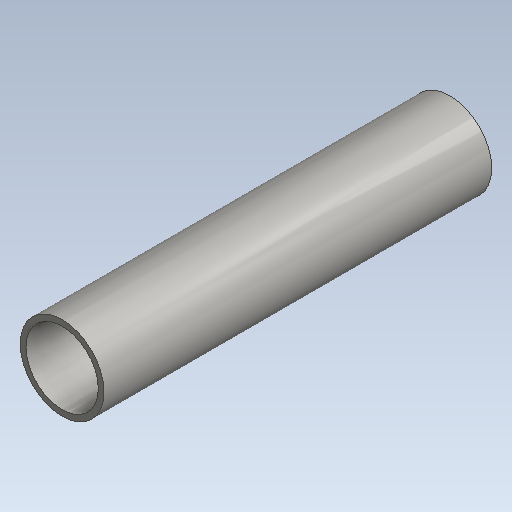
# Autodesk Inventor part: OR0G18180
Saved by Autodesk Inventor 2021 (Build 250183000, 183)
## iProperties
Created: 2020-04-29
Part Number: OR0G18180
Material: Steel AISI 4130
Document SubType Name: Modeling
Designer: Hannah
Density: 7.85 g/cm^3
Appearance: Steel
Mass: 245.777 g
Surface Area: 288.803 cm^2
Volume: 31.3091 cm^3
Catalog Web Link: https://www.framebuilding.com/ZONA.htm
Description: head tube
Vendor: Ceeway
OD: 32.4
Length: 150.0
Size: [6]
Author: Hannah
Revision Number: -
Autodesk Inventor part; units mm, degrees
ref_plane "YZ Plane" through (0, 0, 0) normal (1, 0, 0) x (0, 1, 0)
ref_plane "XZ Plane" through (0, 0, 0) normal (0, 1, 0) x (-1, 0, 0)
ref_plane "XY Plane" through (0, 0, 0) normal (0, 0, 1) x (1, 0, 0)
sketch "Sketch1" plane through (0, 0, 0) normal (0, 0, 1) x (1, 0, 0)
  circle A0 centre (0, 0) radius 14
  circle A1 centre (0, 0) radius 16.2
  dimension "d0" = 28
  dimension "OD" = 32.4
  constraints: 2 centre point, 2 coincident
  measures "d0" diameter of A0
  measures "OD" diameter of A1
extrude "Extrusion1" add sketch "Sketch1" along normal mid plane 150
body "Solid1"
